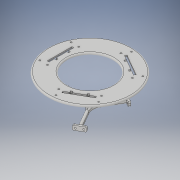
# Autodesk Inventor part: Stewart-Platform-Base-Außenanordnung
Saved by Autodesk Inventor 2018.2 (Build 222227000, 227)
## iProperties
Created: 2018-02-17
Part Number: Stewart-Platform-Base-Außenanordnung
Material: Generisch
Document SubType Name: Modeling
Designer: JochenAlt
Density: 1 g/cm^3
Appearance: Vorgabe
Author: JochenAlt
Autodesk Inventor part; units mm, degrees
ref_plane "YZ Plane" through (0, 0, 0) normal (1, 0, 0) x (0, 1, 0)
ref_plane "XZ Plane" through (0, 0, 0) normal (0, 1, 0) x (-1, 0, 0)
sketch "Skizze1" plane through (0, 0, 0) normal (0, 0, 1) x (1, 0, 0)
  line L0 (0, 95.9835) -> (0, -95.9835) construction
  line L1 (-95.9835, 0) -> (95.9835, 0) construction
  line L2 (-56.4464, 28.85) -> (-43.9464, 28.85) construction
  line L3 (-40.6464, 25.55) -> (-40.6464, -25.55) construction
  line L4 (-43.9464, -28.85) -> (-56.4464, -28.85) construction
  line L5 (-59.7464, -25.55) -> (-59.7464, 25.55) construction
  arc A0 (-56.4464, 28.85) -> (-59.7464, 25.55) centre (-56.4464, 25.55) ccw construction
  arc A1 (-40.6464, 25.55) -> (-43.9464, 28.85) centre (-43.9464, 25.55) ccw construction
  arc A2 (-43.9464, -28.85) -> (-40.6464, -25.55) centre (-43.9464, -25.55) ccw construction
  arc A3 (-59.7464, -25.55) -> (-56.4464, -28.85) centre (-56.4464, -25.55) ccw construction
  circle A4 centre (-56.4464, 25.55) radius 1.3
  circle A5 centre (-43.9464, 25.55) radius 1.3
  circle A6 centre (-56.4464, -25.55) radius 1.3
  circle A7 centre (-43.9464, -25.55) radius 1.3
  line L6 (-46.6464, 20.25) -> (-46.6464, -20.25)
  line L7 (-49.7464, 20.25) -> (-49.7464, -20.25)
  line L8 (-49.7464, 20.25) -> (-46.6464, 20.25)
  line L9 (-49.7464, -20.25) -> (-46.6464, -20.25)
  line L10 (-49.7464, 0.8) -> (-46.6464, 0.8)
  line L11 (-49.7464, -0.8) -> (-46.6464, -0.8)
  line L12 (-46.6464, 11.55) -> (-43.6304, 11.55)
  line L13 (-43.6304, 11.55) -> (-43.6304, 8.75)
  line L14 (-43.6304, 8.75) -> (-46.6464, 8.75)
  line L15 (-46.6464, -8.75) -> (-43.6304, -8.75)
  line L16 (-43.6304, -8.75) -> (-43.6304, -11.55)
  line L17 (-43.6304, -11.55) -> (-46.6464, -11.55)
  line L18 (-43.9464, 29.15) -> (-56.4464, 29.15)
  arc A8 (-56.4464, 29.15) -> (-60.0464, 25.55) centre (-56.4464, 25.55) ccw
  line L19 (-60.0464, 25.55) -> (-60.0464, -25.55)
  arc A9 (-60.0464, -25.55) -> (-56.4464, -29.15) centre (-56.4464, -25.55) ccw
  line L20 (-56.4464, -29.15) -> (-43.9464, -29.15)
  arc A10 (-43.9464, -29.15) -> (-40.3464, -25.55) centre (-43.9464, -25.55) ccw
  line L21 (-40.3464, -25.55) -> (-40.3464, 25.55)
  arc A11 (-40.3464, 25.55) -> (-43.9464, 29.15) centre (-43.9464, 25.55) ccw
  line L22 (-62.1774, -28.8235) -> (-59.5724, -27.3356) construction
  line L23 (-37.3464, 0) -> (-40.3464, 0) construction
  circle A12 centre (0, 0) radius 37.3464
  circle A13 centre (0, 0) radius 68.5597
  line L24 (-62.4591, 28.2716) -> (-59.7261, 27.0345) construction
  line L25 (-43.6304, -10.15) -> (-5.8601, -10.15) construction
  line L26 (6.3855, -31.3601) -> (-5.8601, -10.15) construction
  line L27 (-39.3464, -10.15) -> (-39.3464, -68.15) construction
  line L28 (10.8831, -39.15) -> (-39.3464, -68.15) construction
  line L29 (-40.3464, -19.95) -> (-46.6464, -19.95)
  line L30 (-40.3464, 19.95) -> (-46.6464, 19.95)
  arc A14 (47.2179, -23.4837) -> (42.3002, -22.166) centre (44.1002, -25.2837) ccw
  circle A15 centre (44.1002, -25.2837) radius 1.3
  line L31 (42.3002, -22.166) -> (-1.9537, -47.716)
  line L32 (37.4504, -24.966) -> (40.6004, -30.422)
  line L33 (31.8178, -32.0101) -> (33.3258, -34.622)
  line L34 (29.3929, -33.4101) -> (31.8178, -32.0101)
  line L35 (30.9009, -36.022) -> (29.3929, -33.4101)
  line L36 (5.7862, -50.522) -> (40.8602, -30.272)
  line L37 (42.4102, -32.9567) -> (40.8602, -30.272)
  line L38 (7.3362, -53.2067) -> (42.4102, -32.9567)
  line L39 (25.566, -42.6817) -> (24.016, -39.997)
  line L40 (24.1804, -43.4817) -> (22.6304, -40.797)
  line L41 (11.8126, -43.5601) -> (14.2375, -42.1601)
  line L42 (14.2375, -42.1601) -> (15.7455, -44.772)
  line L43 (13.3206, -46.172) -> (11.8126, -43.5601)
  line L44 (2.896, -44.916) -> (6.046, -50.372)
  line L45 (7.3362, -53.2067) -> (5.7862, -50.522)
  arc A16 (-1.9537, -47.716) -> (-3.2714, -52.6337) centre (-0.1537, -50.8337) ccw
  circle A17 centre (-0.1537, -50.8337) radius 1.3
  line L46 (-3.2714, -52.6337) -> (2.9786, -63.459)
  circle A18 centre (50.3502, -36.109) radius 1.3
  arc A19 (52.1502, -39.2267) -> (53.4679, -34.309) centre (50.3502, -36.109) ccw
  line L47 (7.8963, -64.7767) -> (52.1502, -39.2267)
  circle A20 centre (6.0963, -61.659) radius 1.3
  arc A21 (2.9786, -63.459) -> (7.8963, -64.7767) centre (6.0963, -61.659) ccw
  line L48 (53.4679, -34.309) -> (47.2179, -23.4837)
  arc A22 (-3.2714, 52.6337) -> (-1.9537, 47.716) centre (-0.1537, 50.8337) ccw
  circle A23 centre (-0.1537, 50.8337) radius 1.3
  line L49 (-1.9537, 47.716) -> (42.3002, 22.166)
  line L50 (2.896, 44.916) -> (6.046, 50.372)
  line L51 (11.8126, 43.5601) -> (13.3206, 46.172)
  line L52 (14.2375, 42.1601) -> (11.8126, 43.5601)
  line L53 (15.7455, 44.772) -> (14.2375, 42.1601)
  line L54 (40.8602, 30.272) -> (5.7862, 50.522)
  line L55 (7.3362, 53.2067) -> (5.7862, 50.522)
  line L56 (42.4102, 32.9567) -> (7.3362, 53.2067)
  line L57 (24.1804, 43.4817) -> (22.6304, 40.797)
  line L58 (25.566, 42.6817) -> (24.016, 39.997)
  line L59 (31.8178, 32.0101) -> (29.3929, 33.4101)
  line L60 (29.3929, 33.4101) -> (30.9009, 36.022)
  line L61 (33.3258, 34.622) -> (31.8178, 32.0101)
  line L62 (37.4504, 24.966) -> (40.6004, 30.422)
  line L63 (42.4102, 32.9567) -> (40.8602, 30.272)
  arc A24 (42.3002, 22.166) -> (47.2179, 23.4837) centre (44.1002, 25.2837) ccw
  circle A25 centre (44.1002, 25.2837) radius 1.3
  line L64 (47.2179, 23.4837) -> (53.4679, 34.309)
  circle A26 centre (6.0963, 61.659) radius 1.3
  arc A27 (7.8963, 64.7767) -> (2.9786, 63.459) centre (6.0963, 61.659) ccw
  line L65 (52.1502, 39.2267) -> (7.8963, 64.7767)
  circle A28 centre (50.3502, 36.109) radius 1.3
  arc A29 (53.4679, 34.309) -> (52.1502, 39.2267) centre (50.3502, 36.109) ccw
  line L66 (2.9786, 63.459) -> (-3.2714, 52.6337)
  point P0 (0, 2)
  point P1 (0, -2)
  point P2 (-40.3464, -21.4)
  point P3 (-40.3464, 21.4)
  point P4 (20.1732, -34.941)
  point P5 (38.7062, -24.241)
  point P6 (1.6403, -45.641)
  point P7 (30.6054, -32.7101)
  point P8 (53.4595, -37.9234)
  point P9 (6.4505, -65.2416)
  point P10 (20.1732, 34.941)
  point P11 (1.6403, 45.641)
  point P12 (38.7062, 24.241)
  point P13 (13.0251, 42.8601)
  point P14 (6.1129, 65.259)
  point P15 (53.2756, 38.2071)
  dimension "d43" = 137.1193
  dimension "d1" = 57.7
  dimension "d2" = 19.1
  dimension "d3" = 3.3
  dimension "d5" = 2.6
  dimension "d6" = 6
  dimension "d7" = 3.1
  dimension "d9" = 1.6
  dimension "d10" = 2.984
  dimension "d11" = 2.8
  dimension "d12" = 17.5
  dimension "d21" = 0.3
  dimension "d22" = 3
  dimension "d34" = 3
  dimension "d35" = 3
  dimension "d40" = 1
  dimension "d42" = 58
  dimension "d105" = 360
  dimension "d107" = 40.5
  dimension "d108" = 0.3
  dimension "d109" = 1
  constraints: 124 end point, 38 point on circle, 28 centre point, 23 point on line, 13 coincident, 11 horizontal, 8 tangent, 6 equal radius, 6 perpendicular, 4 midpoint, 4 parallel, 2 line through centre, 2 vertical, 1 collinear, 1 horizontal alignment, 257 other
  measures "d1" distance between parallel lines of L4 L2
  measures "d2" distance between parallel lines of L3 L5
  measures "d3" radius of A0
  measures "d5" diameter of A4
  measures "d9" distance between parallel lines of L11 L10
  measures "d10" distance between parallel lines of L3 L13
  measures "d11" distance between parallel lines of L14 L12
  measures "d12" distance between parallel lines of L15 L14
  measures "d21" distance between parallel lines of L19 L5
  measures "d22" distance of L22.end L22.start
  measures "d34" distance of L23.start L23.end
  measures "d35" distance of L24.start L24.end
  measures "d40" distance between parallel lines of L21 L27
  measures "d42" distance from line of L25 L27.end
  measures "d107" distance between parallel lines of L8 L9
  measures "d108" distance between parallel lines of L29 L9
  measures "d109" distance between parallel lines of L28 L31
extrude "Extrusion5" add sketch "Skizze1" along normal blind 4 contours L8 L7 L9 L6 L29 L21 A10 L20 A9 L19 A8 L18 A11 L30 | L30 L21 L29 L6 L17 L16 L15 L14 L13 L12 | A13 | L48 A19 L47 A21 L46 A16 L31 L44 L36 L45 L38 L37 L32 A14 | L32 L36 L33 L34 L35 L42 L41 L43 L44 L31 | L66 A27 L65 A29 L64 A24 L49 L62 L54 L63 L56 L55 L50 A22 | L50 L54 L51 L52 L53 L60 L59 L61 L62 L49
extrude "Extrusion4" cut sketch "Skizze1" along normal blind 2 contours L8 L7 L9 L6 L29 L21 A10 L20 A9 L19 A8 L18 A11 L30 | L48 A19 L47 A21 L46 A16 L31 L44 L36 L45 L38 L37 L32 A14 | L66 A27 L65 A29 L64 A24 L49 L62 L54 L63 L56 L55 L50 A22
ref_plane "Arbeitsebene2" through (0, 0, -41.8) normal (0, 0, 1) x (1, 0, 0)
sketch "Skizze6" plane through (0, 0, -41.8) normal (0, 0, 1) x (1, 0, 0)
  line L0 (-46.6464, 8.75) -> (-46.6464, -8.75) construction
  line L1 (-46.6464, -8.75) -> (-43.6304, -8.75) construction
  line L2 (-43.6304, -8.75) -> (-43.6304, -11.55) construction
  line L3 (-43.6304, -11.55) -> (-46.6464, -11.55) construction
  line L4 (-46.6464, -11.55) -> (-46.6464, -20.25) construction
  line L5 (-46.6464, -20.25) -> (-49.7464, -20.25) construction
  line L6 (-49.7464, -20.25) -> (-49.7464, 20.25) construction
  line L7 (-46.6464, 20.25) -> (-46.6464, 11.55) construction
  line L8 (-46.6464, 11.55) -> (-43.6304, 11.55) construction
  line L9 (-43.6304, 11.55) -> (-43.6304, 8.75) construction
  line L10 (-43.6304, 8.75) -> (-46.6464, 8.75) construction
  line L11 (-49.7464, 20.25) -> (-46.6464, 20.25) construction
  circle A0 centre (-43.9464, -25.55) radius 1.3 construction
  circle A1 centre (-56.4464, -25.55) radius 1.3 construction
  circle A2 centre (-43.9464, 25.55) radius 1.3 construction
  circle A3 centre (-56.4464, 25.55) radius 1.3 construction
  circle A4 centre (0, 0) radius 37.3464 construction
  circle A5 centre (0, 0) radius 68.5597 construction
  line L12 (-46.6464, -8.75) -> (-46.6464, 8.75)
  line L13 (-46.6464, -8.75) -> (-43.6304, -8.75)
  line L14 (-46.6464, 8.75) -> (-46.6464, -8.75) projected
  line L15 (-95.2478, 0) -> (95.2478, 0) construction
  line L16 (0, 95.2478) -> (0, -95.2478) construction
  line L17 (-43.6304, 8.75) -> (-43.6304, 2)
  line L18 (-43.6304, -2) -> (-43.6304, -8.75)
  line L19 (0, 0) -> (-8.9019, -15.4186) construction
  line L20 (0, 0) -> (-9.1171, 15.7912) construction
  arc A6 (-2.7017, -4.6795) -> (-12.7017, -2) centre (-12.7017, -22) ccw
  arc A7 (-12.7017, 2) -> (-2.7017, 4.6795) centre (-12.7017, 22) ccw
  line L21 (-2.7017, -4.6795) -> (0, -6.2393)
  line L22 (-2.7017, 4.6795) -> (0, 6.2393)
  line L23 (-43.6304, -2) -> (-12.7017, -2)
  line L24 (-43.6304, 2) -> (-12.7017, 2)
  line L25 (-43.6304, 8.75) -> (-46.6464, 8.75) projected
  line L26 (-46.6464, 8.75) -> (-43.6304, 8.75)
  arc A8 (0, 1.65) -> (0, -1.65) centre (0, 0) ccw
  line L27 (0, -6.2393) -> (0, -1.65)
  line L28 (0, 1.65) -> (0, 6.2393)
  point P0 (-33.3674, -0.8)
  dimension "d73" = 120
  dimension "d89" = 20
  dimension "d90" = 4
  dimension "d91" = 3.3
  constraints: 26 end point, 6 point on circle, 6 point on line, 5 perpendicular, 4 tangent, 3 centre point, 2 parallel, 1 coincident, 1 collinear, 1 symmetric about line, 1 vertical, 3 other
  measures "d73" angle of L20 L19
  measures "d89" radius of A7
  measures "d90" distance between parallel lines of L23 L24
  measures "d91" diameter of A8
extrude "Extrusion9" add sketch "Skizze6" against normal blind 7.1 separate body
sketch "Skizze7" plane through (-46.6464, -8.75, -41.8) normal (-1, 0, 0) x (0, 0, -1)
  circle A0 centre (3.8, -3.7) radius 1.3
  circle A1 centre (3.8, -13.8) radius 1.3
  line L0 (0, -17.5) -> (0, 0) construction
  line L1 (0, -8.75) -> (7.1, -8.75) construction
  line L2 (7.1, 0) -> (7.1, -17.5) construction
  point P0 (-41.8, -8.75)
  dimension "d76" = 2.6
  dimension "d77" = 10.1
  dimension "d88" = 3.3
  constraints: 2 centre point, 2 end point, 2 midpoint, 1 equal radius, 1 symmetric about line
  measures "d76" diameter of A1
  measures "d77" distance of A0.centre A1.centre
  measures "d88" distance from line of A0.centre L2
extrude "Extrusion10" cut sketch "Skizze7" against normal blind 10 bodies 1 2
pattern_circular "Runde Anordnung5" count 3 over 360 about axis through (0, 0, -10) along (0, 0, 1) of "Extrusion10", "Extrusion9" bodies 2
fillet "Rundung1" radius 2 30 edges at (-2.7017, -4.6795, -41.8) (-28.1661, -2, -41.8) (12.351, -25.3925, -41.8) (-2.7017, 4.6795, -41.8) (12.351, 25.3925, -41.8) (-28.1661, 2, -41.8) (15.8151, 23.3925, -41.8) (15.8151, -23.3925, -41.8) (5.4034, 0, -41.8) (-2.7017, -4.6795, -48.9) (-28.1661, -2, -48.9) (12.351, -25.3925, -48.9) (15.8151, -23.3925, -48.9) (15.8151, 23.3925, -48.9) (5.4034, 0, -48.9) (-45.1384, 8.75, -48.9) (-45.1384, -8.75, -48.9) (14.9915, 43.466, -48.9) (30.1469, 34.716, -48.9) (30.1469, 34.716, -41.8) (14.9915, 43.466, -41.8) (-45.1384, 8.75, -41.8) (-45.1384, -8.75, -41.8) (14.9915, -43.466, -41.8) (14.9915, -43.466, -48.9) (30.1469, -34.716, -41.8) (30.1469, -34.716, -48.9) (12.351, 25.3925, -48.9) (-28.1661, 2, -48.9) (-2.7017, 4.6795, -48.9)
fillet "Rundung2" radius 2 4 edges at (-68.5597, 0, 4) (-68.5597, 0, 0) (-37.3464, 0, 0) (-37.3464, 0, 4)
equation "\"d22\" = d20"
equation "\"d35\" = d34"
equation "\"d44\" = d21"
equation "\"d20\" = 3"
